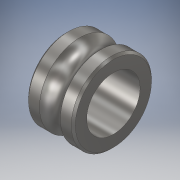
# Autodesk Inventor part: Bearings - Inner Race
Saved by Autodesk Inventor 2019 (Build 230136000, 136)
## iProperties
Created: 2020-12-03
Part Number: Bearings - Inner Race
Material: Stainless Steel
Document SubType Name: Modeling
Designer: Anass Hamdi
Density: 8 g/cm^3
Appearance: Semi-Polished
Author: Anass Hamdi
Autodesk Inventor part; units mm, degrees
ref_plane "YZ Plane" through (0, 0, 0) normal (1, 0, 0) x (0, 1, 0)
ref_plane "XZ Plane" through (0, 0, 0) normal (0, 1, 0) x (-1, 0, 0)
ref_plane "XY Plane" through (0, 0, 0) normal (0, 0, 1) x (1, 0, 0)
sketch "Sketch1" plane through (0, 0, 0) normal (0, 0, 1) x (1, 0, 0)
  line L0 (0, 0) -> (0, -4) construction
  line L1 (-3.5, -4) -> (3.5, -4)
  line L2 (3.5, -4) -> (3.5, -6)
  line L3 (-3.5, -4) -> (-3.5, -6)
  line L4 (-4.9, 0) -> (4.9, 0) projected
  line L5 (0, -6) -> (0, -7.25) construction
  arc A0 (1.5612, -6) -> (-1.5612, -6) centre (0, -7.25) ccw
  line L6 (-3.5, -6) -> (-1.5612, -6)
  line L7 (1.5612, -6) -> (3.5, -6)
  dimension "d0" = 4
  dimension "d1" = 7
  dimension "d2" = 2
  dimension "d10" = 1.25
  dimension "d11" = 4
  constraints: 14 end point, 3 horizontal, 3 vertical, 2 point on circle, 1 centre point, 1 coincident, 1 perpendicular
  measures "d0" distance of L0.start L0.end
  measures "d1" distance of L1.start L1.end
  measures "d2" distance of L1.end L2.end
  measures "d10" distance of L5.start L5.end
  measures "d11" diameter of A0
revolve "Revolution1" add sketch "Sketch1" angle 360 about axis through (-10, 0, 0) along (1, 0, 0)
chamfer "Chamfer1" distance 0.3 angle 45 2 edges at (-3.5, 6, 0) (3.5, 6, 0)
body "Solid1"
